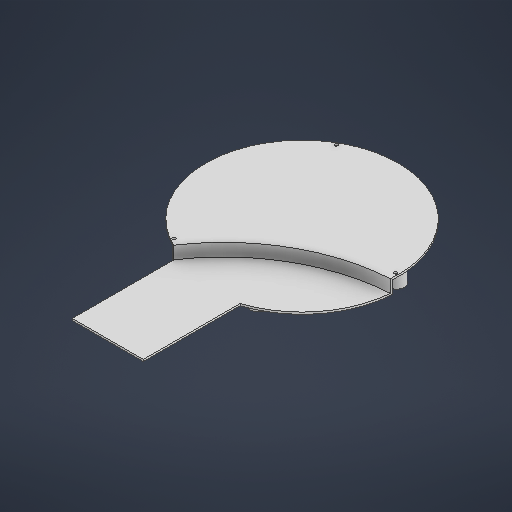
# Autodesk Inventor part: bottom_replacement_housing_bottom
Saved by Autodesk Inventor 2026 (Build 300175000, 175)
## iProperties
Created: 2025-05-12
Part Number: bottom_replacement_housing_bottom
Material: Generic
Document SubType Name: Sheet Metal
Designer: Paul Juschitz
Density: 1 g/cm^3
Sheet Metal Rule: Default_mm
Appearance: Default
Author: Paul Juschitz
Autodesk Inventor part; units mm, degrees
ref_plane "YZ Plane" through (0, 0, 0) normal (1, 0, 0) x (0, 1, 0)
ref_plane "XZ Plane" through (0, 0, 0) normal (0, 1, 0) x (-1, 0, 0)
ref_plane "XY Plane" through (0, 0, 0) normal (0, 0, 1) x (1, 0, 0)
derived "m2m_shell.ipt"
sketch "Sketch1" plane through (0, 0, 0) normal (0, 1, 0) x (-1, 0, 0)
  circle A0 centre (36.9504, 64) radius 1.25
  circle A1 centre (36.9504, -64) radius 1.25
  circle A2 centre (-73.9008, 0) radius 1.25
  line L0 (36.9504, 64) -> (36.9504, -64) construction
  line L1 (36.9504, -64) -> (-73.9008, 0) construction
  line L2 (-73.9008, 0) -> (36.9504, 64) construction
  line L3 (-73.9008, 0) -> (36.9504, 0)
  line L4 (36.9504, 64) -> (-18.4752, -32)
  line L5 (36.9504, -64) -> (-18.4752, 32)
  line L6 (0, -136.5769) -> (0, 186.0374) construction
  circle A3 centre (0, 0) radius 76
  dimension "bottom_screwhole_diameter" = 2.5
  dimension "bottom_screwhole_spacing" = 128
  dimension "bottom_screwhole_angle" = 30
  dimension "d6" = 152
  constraints: 14 end point, 4 centre point, 3 midpoint, 2 coincident, 2 equal length, 2 equal radius, 2 point on line, 1 vertical, 2 other
  measures "bottom_screwhole_diameter" diameter of A0
  measures "bottom_screwhole_spacing" distance of L0.end L1.end
  measures "bottom_screwhole_angle" angle of L6 L5
  measures "d6" diameter of A3
extrude "Extrusion1" add sketch "Sketch1" along normal blind 1.5
sketch "Sketch2" plane through (0, 1.5, 0) normal (0, 1, 0) x (1, 0, 0)
  circle A0 centre (0, 0) radius 76 construction
  arc A1 (75.7514, -6.1418) -> (-32.5568, -68.6736) centre (84.2268, -145.885) ccw
  line L0 (-76, 0) -> (76, 0) construction
  line L1 (84.2268, -145.885) -> (0, 0) construction
  circle A2 centre (-36.9504, -64) radius 1.25 projected
  arc A3 (-32.5568, -68.6736) -> (75.7514, -6.1418) centre (0, 0) ccw
  dimension "bottom_cutout_radius" = 140
  dimension "bottom_cutout_angle" = 120
  dimension "bottom_cutout_clearance" = 5
  constraints: 10 point on circle, 4 end point, 2 centre point, 1 concentric, 1 horizontal, 1 line through centre
  measures "bottom_cutout_radius" radius of A1
  measures "bottom_cutout_angle" angle of L0 L1
extrude "Extrusion2" cut sketch "Sketch2" against normal through all contours A3 A1
sketch "Sketch3" plane through (0, 0, 0) normal (0, -1, 0) x (1, 0, 0)
  arc A0 (-32.5568, 68.6736) -> (75.7514, 6.1418) centre (84.2268, 145.885) ccw projected
  arc A1 (-32.5568, 68.6736) -> (75.7514, 6.1418) centre (0, 0) ccw construction
  circle A2 centre (73.9008, 0) radius 1.25 construction
  circle A3 centre (-36.9504, 64) radius 1.25 construction
  arc A4 (75.8587, 4.6327) -> (75.7514, 6.1418) centre (0, 0) ccw
  arc A5 (-33.9173, 68.0119) -> (75.8587, 4.6327) centre (84.2268, 145.885) ccw
  arc A6 (-32.5568, 68.6736) -> (-33.9173, 68.0119) centre (0, 0) ccw
  dimension "d16" = 1.5
  constraints: 8 point on circle, 3 centre point, 3 coincident
  measures "d16" radial gap between concentric circles of A5 A0
extrude "Extrusion3" add sketch "Sketch3" along normal blind 10
ref_plane "bottom extension plane" through (0, -8.5, 0) normal (0, -1, 0) x (1, 0, 0)
sketch "Sketch4" plane through (0, -8.5, 0) normal (0, -1, 0) x (1, 0, 0)
  arc A0 (-32.5568, 68.6736) -> (75.7514, 6.1418) centre (84.2268, 145.885) ccw projected
  arc A1 (-32.5568, 68.6736) -> (75.7514, 6.1418) centre (0, 0) ccw construction
  circle A2 centre (0, 0) radius 76 construction
  line L0 (-32.5568, 68.6736) -> (-32.5568, 148.6736)
  line L1 (-32.5568, 148.6736) -> (23.4432, 148.6736)
  line L2 (23.4432, 148.6736) -> (23.4432, 72.2939)
  arc A3 (75.7514, 6.1418) -> (23.4432, 72.2939) centre (0, 0) ccw
  dimension "bottom_extension_outset" = 80
  dimension "bottom_core_outer_width" = 56
  constraints: 6 end point, 2 perpendicular, 2 point on circle, 1 centre point, 1 concentric, 1 vertical, 6 other
  measures "bottom_extension_outset" distance of L0.start L0.end
  measures "bottom_core_outer_width" distance of L0.end L1.end
extrude "Extrusion5" add sketch "Sketch4" along normal up to surface (1.5 mm away)
sketch "Sketch5" plane through (0, 0, 0) normal (0, -1, 0) x (1, 0, 0)
  arc A0 (-33.9173, 68.0119) -> (75.8587, 4.6327) centre (0, 0) ccw construction
  circle A1 centre (67.3954, -6.9231) radius 6.25
  circle A2 centre (73.9008, 0) radius 1.25 projected
  circle A3 centre (27.4105, 61.9574) radius 6.25
  circle A4 centre (-50.4547, 45.2149) radius 6.25
  circle A5 centre (-58.5933, -34.0131) radius 6.25
  circle A6 centre (14.2421, -66.2361) radius 6.25
  dimension "bottom_foot_OD" = 12.5
  dimension "bottom_foot_inset" = 2
  dimension "d30" = 2
  dimension "d33" = 360
  constraints: 5 centre point, 1 coincident, 11 other
  measures "bottom_foot_OD" diameter of A1
extrude "Extrusion6" add sketch "Sketch5" along normal blind 11 contours A1 | A4 | A5 | A6
sketch "Sketch6" plane through (67.3954, -11, -6.9231) normal (0, -1, 0) x (1, 0, 0)
  circle A0 centre (0, 0) radius 6.25 projected
  circle A1 centre (-53.1533, -59.3131) radius 6.25 projected
  circle A2 centre (-125.9886, -27.0901) radius 6.25 projected
  circle A3 centre (-117.8501, 52.1379) radius 6.25 projected
  circle A4 centre (0, 0) radius 5.25
  circle A5 centre (-53.1533, -59.3131) radius 5.25
  circle A6 centre (-125.9886, -27.0901) radius 5.25
  circle A7 centre (-117.8501, 52.1379) radius 5.25
  point P0 (-67.3954, 6.9231)
  dimension "d37" = 1
  constraints: 4 centre point, 4 coincident, 3 equal radius
  measures "d37" radial gap between concentric circles of A3 A7
extrude "Extrusion7" add sketch "Sketch6" along normal blind 1
sketch "Sketch7" plane through (0, -10, 0) normal (0, -1, 0) x (1, 0, 0)
  circle A0 centre (27.4105, 61.9574) radius 6.25 projected
  point P0 (0, 0)
extrude "Extrusion8" add sketch "Sketch7" along normal blind 2
sketch "Sketch8" plane through (27.4105, -12, 61.9574) normal (0, -1, 0) x (1, 0, 0)
  circle A0 centre (0, 0) radius 6.25 projected
  circle A1 centre (0, 0) radius 5.25
  point P0 (-27.4105, -61.9574)
  dimension "d42" = 1
  constraints: 1 centre point, 1 coincident
  measures "d42" radial gap between concentric circles of A0 A1
extrude "Extrusion9" add sketch "Sketch8" along normal blind 1
equation "\"bottom_screwhole_diameter\" = m2m_shell_bottom_screwhole_ID"
equation "\"d6\" = 2 * m2m_bottom_radius_lower"
equation "\"d16\" = bottom_material_thickness"
equation "\"BendRadius\" = Thickness"
equation "\"BendReliefWidth\" = Thickness"
equation "\"BendReliefDepth\" = 0.5 * Thickness"
equation "\"CornerReliefSize\" = 4 * Thickness"
equation "\"MinimumRemnant\" = 2 * Thickness"
equation "\"TransitionRadius\" = BendRadius"
equation "\"JacobiRadiusSize\" = BendRadius"
equation "\"GapSize\" = Thickness"
equation "\"d19\" = -bottom_material_thickness"
equation "\"m2m_shell_bottom_screwhole_ID\" = 2.5"
equation "\"m2m_bottom_radius_lower\" = 76"
equation "\"bottom_material_thickness\" = 1.5"
equation "\"Thickness\" = 0.5"
body "Solid1"
